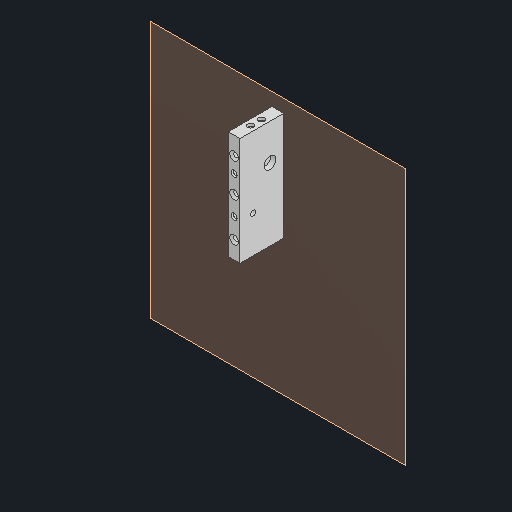
# Autodesk Inventor part: middle_gear_holder
Saved by Autodesk Inventor 2023 (Build 270158000, 158)
## iProperties
Created: 2024-04-23
Part Number: middle_gear_holder
Material: Generic
Document SubType Name: Modeling
Designer: szymo
Density: 1 g/cm^3
Appearance: Default
Author: szymo
Autodesk Inventor part; units mm, degrees
ref_plane "YZ Plane" through (0, 0, 0) normal (1, 0, 0) x (0, 1, 0)
ref_plane "XZ Plane" through (0, 0, 0) normal (0, 1, 0) x (-1, 0, 0)
ref_plane "XY Plane" through (0, 0, 0) normal (0, 0, 1) x (1, 0, 0)
ref_plane "Work Plane1" through (0, 0, 0) normal (0, 0, 1) x (1, 0, 0)
ref_plane "Work Plane2" through (-89, -40.3889, 33.5) normal (0, 0, 1) x (1, 0, 0)
sketch "Sketch1" plane through (0, 0, 0) normal (0, 0, 1) x (1, 0, 0)
  line L0 (23.5, 88.5) -> (-23.5, 88.5) projected
  line L1 (-23.5, 88.5) -> (-23.5, 36.5) projected
  line L2 (-26.5, 33.5) -> (-89, 33.5) projected
  line L3 (-89, 33.5) -> (-89, -72.5) projected
  line L4 (-89, -72.5) -> (-77, -72.5) projected
  line L5 (-74, -75.5) -> (-74, -93.5) projected
  line L6 (-74, -93.5) -> (74, -93.5) projected
  line L7 (74, -93.5) -> (74, -75.5) projected
  line L8 (77, -72.5) -> (89, -72.5) projected
  line L9 (89, -72.5) -> (89, 33.5) projected
  line L10 (89, 33.5) -> (26.5, 33.5) projected
  line L11 (23.5, 36.5) -> (23.5, 88.5) projected
  line L12 (-4.5, 81.5) -> (-4.5, 36.5) projected
  line L13 (-7.5, 33.5) -> (-13.5, 33.5) projected
  line L14 (-16.5, 36.5) -> (-16.5, 81.5) projected
  line L15 (7.5, 84.5) -> (13.5, 84.5) projected
  line L16 (16.5, 81.5) -> (16.5, 36.5) projected
  line L17 (13.5, 33.5) -> (7.5, 33.5) projected
  line L18 (4.5, 36.5) -> (4.5, 81.5) projected
  line L19 (-13.5, 84.5) -> (-7.5, 84.5) projected
  line L20 (-4.5, 88.5) -> (4.5, 88.5)
  line L21 (4.5, 88.5) -> (4.5, 5.75)
  line L22 (4.5, 5.75) -> (-4.5, 5.75)
  line L23 (-4.5, 5.75) -> (-4.5, 88.5)
  line L24 (-32.2, 4.75) -> (-59.9, 4.75)
  arc A0 (13.5, 33.5) -> (16.5, 36.5) centre (13.5, 36.5) ccw projected
  arc A1 (4.5, 36.5) -> (7.5, 33.5) centre (7.5, 36.5) ccw projected
  arc A2 (7.5, 84.5) -> (4.5, 81.5) centre (7.5, 81.5) ccw projected
  arc A3 (16.5, 81.5) -> (13.5, 84.5) centre (13.5, 81.5) ccw projected
  arc A4 (-4.5, 81.5) -> (-7.5, 84.5) centre (-7.5, 81.5) ccw projected
  arc A5 (-7.5, 33.5) -> (-4.5, 36.5) centre (-7.5, 36.5) ccw projected
  arc A6 (-16.5, 36.5) -> (-13.5, 33.5) centre (-13.5, 36.5) ccw projected
  arc A7 (-13.5, 84.5) -> (-16.5, 81.5) centre (-13.5, 81.5) ccw projected
  arc A8 (-26.5, 33.5) -> (-23.5, 36.5) centre (-26.5, 36.5) ccw projected
  arc A9 (-74, -75.5) -> (-77, -72.5) centre (-77, -75.5) ccw projected
  arc A10 (77, -72.5) -> (74, -75.5) centre (77, -75.5) ccw projected
  arc A11 (23.5, 36.5) -> (26.5, 33.5) centre (26.5, 36.5) ccw projected
  circle A12 centre (21.5, -85.5) radius 1.8 projected
  circle A13 centre (-64.5, -85.5) radius 1.8 projected
  circle A14 centre (83.4, -16.3889) radius 1.8 projected
  circle A15 centre (-83.4, -19.2889) radius 1.8 projected
  circle A16 centre (-21.5, -85.5) radius 1.8 projected
  circle A17 centre (64.5, -85.5) radius 1.8 projected
  circle A18 centre (-56.0375, 15.0937) radius 1.0065 projected
  circle A19 centre (39.125, 4.3375) radius 1.0065 projected
  circle A20 centre (-72.95, 4.275) radius 1.0065 projected
  circle A21 centre (39.125, 25.9125) radius 1.0065 projected
  circle A22 centre (72.95, 12.275) radius 1.0065 projected
  circle A23 centre (86, 30.5) radius 1.0065 projected
  circle A24 centre (-86, 30.5) radius 1.0065 projected
  circle A25 centre (-39.125, 12.3375) radius 1.0065 projected
  circle A26 centre (-72.95, 25.975) radius 1.0065 projected
  circle A27 centre (-72.95, 12.275) radius 1.0065 projected
  circle A28 centre (-39.125, 25.9125) radius 1.0065 projected
  circle A29 centre (-86, 7.75) radius 1.0065 projected
  circle A30 centre (86, 7.75) radius 1.0065 projected
  circle A31 centre (72.95, 25.975) radius 1.0065 projected
  circle A32 centre (39.125, 12.3375) radius 1.0065 projected
  circle A33 centre (-39.125, 4.3375) radius 1.0065 projected
  circle A34 centre (72.95, 4.275) radius 1.0065 projected
  circle A35 centre (56.0375, 15.125) radius 1.0065 projected
  circle A36 centre (78, -67.1725) radius 1.2295 projected
  circle A37 centre (-24.1, -73.1) radius 1.2295 projected
  circle A38 centre (24.1, -24.9) radius 1.2295 projected
  circle A39 centre (-42.5, -43.2802) radius 1.2295 projected
  circle A40 centre (-79, -42.3889) radius 1.2295 projected
  circle A41 centre (-19.5, 28.875) radius 1.2295 projected
  circle A42 centre (19.5, 9.55) radius 1.2295 projected
  circle A43 centre (19.5, 47.3) radius 1.2295 projected
  circle A44 centre (-19.5, 47.3) radius 1.2295 projected
  circle A45 centre (0, 74.7) radius 1.2295 projected
  circle A46 centre (-19.4231, 74.8077) radius 1.2295 projected
  circle A47 centre (19.5, 74.7) radius 1.2295 projected
  circle A48 centre (0, 49.05) radius 1.2295 projected
  circle A49 centre (19.5, 28.875) radius 1.2295 projected
  circle A50 centre (0, 19.125) radius 1.2295 projected
  circle A51 centre (-19.5, 9.55) radius 1.2295 projected
  circle A52 centre (-78, -67.1725) radius 1.2295 projected
  circle A53 centre (-24.1, -24.9) radius 1.2295 projected
  circle A54 centre (24.1, -73.1) radius 1.2295 projected
  circle A55 centre (42.5, -42.7745) radius 1.2295 projected
  circle A56 centre (79, -42.3889) radius 1.2295 projected
  line L25 (-71, -46.1649) -> (-65.2254, -46.1649) projected
  arc A57 (-63.098, -51.2802) -> (-65.2254, -46.1649) centre (-65.2254, -49.1649) ccw projected
  line L26 (-63.098, -51.2802) -> (-68.8726, -57.0881) projected
  arc A58 (-74, -54.9729) -> (-68.8726, -57.0881) centre (-71, -54.9729) ccw projected
  line L27 (-74, -54.9729) -> (-74, -49.1649) projected
  arc A59 (-71, -46.1649) -> (-74, -49.1649) centre (-71, -49.1649) ccw projected
  line L28 (-18.5, -8.7315) -> (-18.5, -4.7315) projected
  arc A60 (-15.5, -1.7315) -> (-18.5, -4.7315) centre (-15.5, -4.7315) ccw projected
  line L29 (-15.5, -1.7315) -> (-8.5, -1.7315) projected
  arc A61 (-5.5, -4.7315) -> (-8.5, -1.7315) centre (-8.5, -4.7315) ccw projected
  line L30 (-5.5, -4.7315) -> (-5.5, -8.7315) projected
  arc A62 (-8.5, -11.7315) -> (-5.5, -8.7315) centre (-8.5, -8.7315) ccw projected
  line L31 (-8.5, -11.7315) -> (-15.5, -11.7315) projected
  arc A63 (-18.5, -8.7315) -> (-15.5, -11.7315) centre (-15.5, -8.7315) ccw projected
  line L32 (-62.5563, -19.7315) -> (-38.9437, -19.7315) projected
  arc A64 (-36.8163, -24.8467) -> (-38.9437, -19.7315) centre (-38.9437, -22.7315) ccw projected
  line L33 (-36.8163, -24.8467) -> (-48.6226, -36.7211) projected
  arc A65 (-52.8774, -36.7211) -> (-48.6226, -36.7211) centre (-50.75, -34.6059) ccw projected
  line L34 (-52.8774, -36.7211) -> (-64.6837, -24.8467) projected
  arc A66 (-62.5563, -19.7315) -> (-64.6837, -24.8467) centre (-62.5563, -22.7315) ccw projected
  line L35 (27.5, -54.9729) -> (27.5, -49.1649) projected
  arc A67 (30.5, -46.1649) -> (27.5, -49.1649) centre (30.5, -49.1649) ccw projected
  line L36 (30.5, -46.1649) -> (36.2746, -46.1649) projected
  arc A68 (38.402, -51.2802) -> (36.2746, -46.1649) centre (36.2746, -49.1649) ccw projected
  line L37 (38.402, -51.2802) -> (32.6274, -57.0881) projected
  arc A69 (27.5, -54.9729) -> (32.6274, -57.0881) centre (30.5, -54.9729) ccw projected
  line L38 (10.6273, -24.5614) -> (1.8773, -35.9288) projected
  arc A70 (-2.8773, -35.9288) -> (1.8773, -35.9288) centre (-0.5, -34.0989) ccw projected
  line L39 (-2.8773, -35.9288) -> (-11.6273, -24.5614) projected
  arc A71 (-9.25, -19.7315) -> (-11.6273, -24.5614) centre (-9.25, -22.7315) ccw projected
  line L40 (-9.25, -19.7315) -> (8.25, -19.7315) projected
  arc A72 (10.6273, -24.5614) -> (8.25, -19.7315) centre (8.25, -22.7315) ccw projected
  line L41 (-32.6274, -57.0881) -> (-38.402, -51.2802) projected
  arc A73 (-36.2746, -46.1649) -> (-38.402, -51.2802) centre (-36.2746, -49.1649) ccw projected
  line L42 (-36.2746, -46.1649) -> (-30.5, -46.1649) projected
  arc A74 (-27.5, -49.1649) -> (-30.5, -46.1649) centre (-30.5, -49.1649) ccw projected
  line L43 (-27.5, -49.1649) -> (-27.5, -54.9729) projected
  arc A75 (-32.6274, -57.0881) -> (-27.5, -54.9729) centre (-30.5, -54.9729) ccw projected
  spline S0 degree 3 poles (58.9, 23.725) (58.9, 24.1577) (58.9848, 24.5947) (59.3384, 25.472) (59.607, 25.8253) (60.2494, 26.5053) (60.6866, 26.7292) (61.3735, 27.0327) (61.8092, 27.1082) (62.6877, 27.1429) (63.1304, 27.039) (63.9304, 26.7523) (64.2888, 26.5005) (64.9284, 25.9459) (65.1766, 25.5677) (65.4139, 25.1026) (65.5281, 24.8465) (65.6683, 24.2527) (65.7, 23.9883) (65.7, 23.725) knots 0 0 0 0 0.129822 0.129822 0.282673 0.282673 0.568071 0.568071 1.093785 1.093785 1.85316 1.85316 2.989395 2.989395 4.855548 4.855548 5.876131 5.876131 6.645928 6.645928 6.645928 6.645928 projected
  line L44 (65.7, 23.725) -> (65.7, 14.525) projected
  spline S1 degree 3 poles (65.7, 14.525) (65.7, 14.0923) (65.6152, 13.6553) (65.2616, 12.778) (64.993, 12.4247) (64.3506, 11.7447) (63.9134, 11.5208) (63.2265, 11.2173) (62.7908, 11.1418) (61.9123, 11.1071) (61.4696, 11.211) (60.6696, 11.4977) (60.3112, 11.7495) (59.6716, 12.3041) (59.4234, 12.6823) (59.1861, 13.1474) (59.0719, 13.4035) (58.9317, 13.9973) (58.9, 14.2617) (58.9, 14.525) knots 0 0 0 0 0.129822 0.129822 0.282673 0.282673 0.568071 0.568071 1.093785 1.093785 1.85316 1.85316 2.989395 2.989395 4.855548 4.855548 5.876131 5.876131 6.645928 6.645928 6.645928 6.645928 projected
  line L45 (58.9, 14.525) -> (58.9, 23.725) projected
  line L46 (-36.734, -33.2737) -> (-32.6274, -29.1434) projected
  arc A76 (-27.5, -31.2586) -> (-32.6274, -29.1434) centre (-30.5, -31.2586) ccw projected
  line L47 (-27.5, -31.2586) -> (-27.5, -35.3889) projected
  arc A77 (-30.5, -38.3889) -> (-27.5, -35.3889) centre (-30.5, -35.3889) ccw projected
  line L48 (-30.5, -38.3889) -> (-34.6065, -38.3889) projected
  arc A78 (-36.734, -33.2737) -> (-34.6065, -38.3889) centre (-34.6065, -35.3889) ccw projected
  line L49 (12.1227, -55.4157) -> (2.6549, -43.1158) projected
  line L50 (2.6549, -43.1158) -> (12.1227, -30.8158) projected
  arc A79 (17.5, -32.6457) -> (12.1227, -30.8158) centre (14.5, -32.6457) ccw projected
  line L51 (17.5, -32.6457) -> (17.5, -53.5858) projected
  arc A80 (12.1227, -55.4157) -> (17.5, -53.5858) centre (14.5, -53.5858) ccw projected
  line L52 (74, -31.2586) -> (74, -36.3889) projected
  arc A81 (71, -39.3889) -> (74, -36.3889) centre (71, -36.3889) ccw projected
  line L53 (71, -39.3889) -> (65.8992, -39.3889) projected
  arc A82 (63.7718, -34.2737) -> (65.8992, -39.3889) centre (65.8992, -36.3889) ccw projected
  line L54 (63.7718, -34.2737) -> (68.8726, -29.1434) projected
  arc A83 (74, -31.2586) -> (68.8726, -29.1434) centre (71, -31.2586) ccw projected
  line L55 (-27.5, -4.7315) -> (-27.5, -8.7315) projected
  arc A84 (-30.5, -11.7315) -> (-27.5, -8.7315) centre (-30.5, -8.7315) ccw projected
  line L56 (-30.5, -11.7315) -> (-42.75, -11.7315) projected
  arc A85 (-45.75, -8.7315) -> (-42.75, -11.7315) centre (-42.75, -8.7315) ccw projected
  line L57 (-45.75, -8.7315) -> (-45.75, -4.7315) projected
  arc A86 (-42.75, -1.7315) -> (-45.75, -4.7315) centre (-42.75, -4.7315) ccw projected
  line L58 (-42.75, -1.7315) -> (-30.5, -1.7315) projected
  arc A87 (-27.5, -4.7315) -> (-30.5, -1.7315) centre (-30.5, -4.7315) ccw projected
  line L59 (74, -4.7315) -> (74, -8.7315) projected
  arc A88 (71, -11.7315) -> (74, -8.7315) centre (71, -8.7315) ccw projected
  line L60 (71, -11.7315) -> (58.75, -11.7315) projected
  arc A89 (55.75, -8.7315) -> (58.75, -11.7315) centre (58.75, -8.7315) ccw projected
  line L61 (55.75, -8.7315) -> (55.75, -4.7315) projected
  arc A90 (58.75, -1.7315) -> (55.75, -4.7315) centre (58.75, -4.7315) ccw projected
  line L62 (58.75, -1.7315) -> (71, -1.7315) projected
  arc A91 (74, -4.7315) -> (71, -1.7315) centre (71, -4.7315) ccw projected
  line L63 (62.5563, -66.5) -> (38.9437, -66.5) projected
  arc A92 (36.8163, -61.3848) -> (38.9437, -66.5) centre (38.9437, -63.5) ccw projected
  line L64 (36.8163, -61.3848) -> (48.6226, -49.5104) projected
  arc A93 (52.8774, -49.5104) -> (48.6226, -49.5104) centre (50.75, -51.6256) ccw projected
  line L65 (52.8774, -49.5104) -> (64.6837, -61.3848) projected
  arc A94 (62.5563, -66.5) -> (64.6837, -61.3848) centre (62.5563, -63.5) ccw projected
  line L66 (17.5, -4.7315) -> (17.5, -8.7315) projected
  arc A95 (14.5, -11.7315) -> (17.5, -8.7315) centre (14.5, -8.7315) ccw projected
  line L67 (14.5, -11.7315) -> (7.5, -11.7315) projected
  arc A96 (4.5, -8.7315) -> (7.5, -11.7315) centre (7.5, -8.7315) ccw projected
  line L68 (4.5, -8.7315) -> (4.5, -4.7315) projected
  arc A97 (7.5, -1.7315) -> (4.5, -4.7315) centre (7.5, -4.7315) ccw projected
  line L69 (7.5, -1.7315) -> (14.5, -1.7315) projected
  arc A98 (17.5, -4.7315) -> (14.5, -1.7315) centre (14.5, -4.7315) ccw projected
  line L70 (38.9437, -19.7315) -> (62.5563, -19.7315) projected
  arc A99 (64.6837, -24.8467) -> (62.5563, -19.7315) centre (62.5563, -22.7315) ccw projected
  line L71 (64.6837, -24.8467) -> (52.8774, -36.7211) projected
  arc A100 (48.6226, -36.7211) -> (52.8774, -36.7211) centre (50.75, -34.6059) ccw projected
  line L72 (48.6226, -36.7211) -> (36.8163, -24.8467) projected
  arc A101 (38.9437, -19.7315) -> (36.8163, -24.8467) centre (38.9437, -22.7315) ccw projected
  line L73 (-18.5, -53.5858) -> (-18.5, -32.6457) projected
  arc A102 (-13.1227, -30.8158) -> (-18.5, -32.6457) centre (-15.5, -32.6457) ccw projected
  line L74 (-13.1227, -30.8158) -> (-3.6549, -43.1158) projected
  line L75 (-3.6549, -43.1158) -> (-13.1227, -55.4157) projected
  arc A103 (-18.5, -53.5858) -> (-13.1227, -55.4157) centre (-15.5, -53.5858) ccw projected
  line L76 (-38.9437, -66.5) -> (-62.5563, -66.5) projected
  arc A104 (-64.6837, -61.3848) -> (-62.5563, -66.5) centre (-62.5563, -63.5) ccw projected
  line L77 (-64.6837, -61.3848) -> (-52.8774, -49.5104) projected
  arc A105 (-48.6226, -49.5104) -> (-52.8774, -49.5104) centre (-50.75, -51.6256) ccw projected
  line L78 (-48.6226, -49.5104) -> (-36.8163, -61.3848) projected
  arc A106 (-38.9437, -66.5) -> (-36.8163, -61.3848) centre (-38.9437, -63.5) ccw projected
  line L79 (-58.9, 23.725) -> (-58.9, 14.525) projected
  spline S2 degree 3 poles (-58.9, 14.525) (-58.9, 14.0923) (-58.9848, 13.6553) (-59.3384, 12.778) (-59.607, 12.4247) (-60.2494, 11.7447) (-60.6866, 11.5208) (-61.3735, 11.2173) (-61.8092, 11.1418) (-62.6877, 11.1071) (-63.1304, 11.211) (-63.9304, 11.4977) (-64.2888, 11.7495) (-64.9284, 12.3041) (-65.1766, 12.6823) (-65.4139, 13.1474) (-65.5281, 13.4035) (-65.6683, 13.9973) (-65.7, 14.2617) (-65.7, 14.525) knots 0 0 0 0 0.129822 0.129822 0.282673 0.282673 0.568071 0.568071 1.093785 1.093785 1.85316 1.85316 2.989395 2.989395 4.855548 4.855548 5.876131 5.876131 6.645928 6.645928 6.645928 6.645928 projected
  line L80 (-65.7, 14.525) -> (-65.7, 23.725) projected
  spline S3 degree 3 poles (-65.7, 23.725) (-65.7, 24.1577) (-65.6152, 24.5947) (-65.2616, 25.472) (-64.993, 25.8253) (-64.3506, 26.5053) (-63.9134, 26.7292) (-63.2265, 27.0327) (-62.7908, 27.1082) (-61.9123, 27.1429) (-61.4696, 27.039) (-60.6696, 26.7523) (-60.3112, 26.5005) (-59.6716, 25.9459) (-59.4234, 25.5677) (-59.1861, 25.1026) (-59.0719, 24.8465) (-58.9317, 24.2527) (-58.9, 23.9883) (-58.9, 23.725) knots 0 0 0 0 0.129822 0.129822 0.282673 0.282673 0.568071 0.568071 1.093785 1.093785 1.85316 1.85316 2.989395 2.989395 4.855548 4.855548 5.876131 5.876131 6.645928 6.645928 6.645928 6.645928 projected
  line L81 (-74, -35.3889) -> (-74, -31.2586) projected
  arc A107 (-68.8726, -29.1434) -> (-74, -31.2586) centre (-71, -31.2586) ccw projected
  line L82 (-68.8726, -29.1434) -> (-64.766, -33.2737) projected
  arc A108 (-66.8935, -38.3889) -> (-64.766, -33.2737) centre (-66.8935, -35.3889) ccw projected
  line L83 (-66.8935, -38.3889) -> (-71, -38.3889) projected
  arc A109 (-74, -35.3889) -> (-71, -38.3889) centre (-71, -35.3889) ccw projected
  line L84 (8.25, -66.5) -> (-9.25, -66.5) projected
  arc A110 (-11.6273, -61.6701) -> (-9.25, -66.5) centre (-9.25, -63.5) ccw projected
  line L85 (-11.6273, -61.6701) -> (-2.8773, -50.3027) projected
  arc A111 (1.8773, -50.3027) -> (-2.8773, -50.3027) centre (-0.5, -52.1326) ccw projected
  line L86 (1.8773, -50.3027) -> (10.6273, -61.6701) projected
  arc A112 (8.25, -66.5) -> (10.6273, -61.6701) centre (8.25, -63.5) ccw projected
  line L87 (68.8726, -57.0881) -> (63.098, -51.2802) projected
  arc A113 (65.2254, -46.1649) -> (63.098, -51.2802) centre (65.2254, -49.1649) ccw projected
  line L88 (65.2254, -46.1649) -> (71, -46.1649) projected
  arc A114 (74, -49.1649) -> (71, -46.1649) centre (71, -49.1649) ccw projected
  line L89 (74, -49.1649) -> (74, -54.9729) projected
  arc A115 (68.8726, -57.0881) -> (74, -54.9729) centre (71, -54.9729) ccw projected
  line L90 (-74, -8.7315) -> (-74, -4.7315) projected
  arc A116 (-71, -1.7315) -> (-74, -4.7315) centre (-71, -4.7315) ccw projected
  line L91 (-71, -1.7315) -> (-58.75, -1.7315) projected
  arc A117 (-55.75, -4.7315) -> (-58.75, -1.7315) centre (-58.75, -4.7315) ccw projected
  line L92 (-55.75, -4.7315) -> (-55.75, -8.7315) projected
  arc A118 (-58.75, -11.7315) -> (-55.75, -8.7315) centre (-58.75, -8.7315) ccw projected
  line L93 (-58.75, -11.7315) -> (-71, -11.7315) projected
  arc A119 (-74, -8.7315) -> (-71, -11.7315) centre (-71, -8.7315) ccw projected
  line L94 (27.5, -8.7315) -> (27.5, -4.7315) projected
  arc A120 (30.5, -1.7315) -> (27.5, -4.7315) centre (30.5, -4.7315) ccw projected
  line L95 (30.5, -1.7315) -> (42.75, -1.7315) projected
  arc A121 (45.75, -4.7315) -> (42.75, -1.7315) centre (42.75, -4.7315) ccw projected
  line L96 (45.75, -4.7315) -> (45.75, -8.7315) projected
  arc A122 (42.75, -11.7315) -> (45.75, -8.7315) centre (42.75, -8.7315) ccw projected
  line L97 (42.75, -11.7315) -> (30.5, -11.7315) projected
  arc A123 (27.5, -8.7315) -> (30.5, -11.7315) centre (30.5, -8.7315) ccw projected
  line L98 (32.6274, -29.1434) -> (37.7282, -34.2737) projected
  arc A124 (35.6008, -39.3889) -> (37.7282, -34.2737) centre (35.6008, -36.3889) ccw projected
  line L99 (35.6008, -39.3889) -> (30.5, -39.3889) projected
  arc A125 (27.5, -36.3889) -> (30.5, -39.3889) centre (30.5, -36.3889) ccw projected
  line L100 (27.5, -36.3889) -> (27.5, -31.2586) projected
  arc A126 (32.6274, -29.1434) -> (27.5, -31.2586) centre (30.5, -31.2586) ccw projected
  point P0 (0, 0)
  point P1 (-4.5, 81.5)
  point P2 (-4.5, 36.5)
  point P3 (7.5, 81.5)
  point P4 (13.5, 81.5)
  point P5 (-7.5, 81.5)
  point P6 (-13.5, 81.5)
  dimension "d41" = 1
  constraints: 10 end point, 2 collinear, 2 horizontal, 2 parallel, 1 perpendicular, 1 point on line, 2 other
  measures "d41" distance between parallel lines of L22 L24
extrude "Extrusion1" add sketch "Sketch1" along normal up to surface (33.5 mm away) contours L21 L18 L22 L23 L12 L0 | A45 | A48 | A50
sketch "Sketch2" plane through (4.5, 5.75, 0) normal (1, 0, 0) x (0, 0, -1)
  circle A0 centre (-23.4363, 28.1825) radius 2 projected
  point P0 (0, -5.75)
extrude "Extrusion2" cut sketch "Sketch2" against normal blind 10
sketch "Sketch3" plane through (4.5, 5.75, 0) normal (1, 0, 0) x (0, 0, -1)
  circle A0 centre (-10.5, 55.25) radius 4.5 projected
  point P0 (0, -5.75)
extrude "Extrusion3" cut sketch "Sketch3" against normal blind 4
sketch "Sketch4" plane through (-4.5, 5.75, 0) normal (-1, 0, 0) x (0, 0, 1)
  circle A0 centre (10.5, 55.25) radius 4.5 projected
  point P0 (0, -5.75)
extrude "Extrusion4" cut sketch "Sketch4" against normal blind 4
sketch "Sketch5" plane through (-4.5, 5.75, 33.5) normal (0, 0, 1) x (1, 0, 0)
  line L0 (5, 59.75) -> (5, 50.75) projected
  line L1 (4, 50.75) -> (4, 59.75) projected
  line L2 (9, 26.1825) -> (0, 26.1825) projected
  line L3 (9, 30.1825) -> (0, 30.1825) projected
  line L4 (17, 78.15) -> (-8, 78.15)
  line L5 (-8, 35.85) -> (17, 35.85)
  line L6 (9, 82.75) -> (9, 0) projected
  line L7 (0, 50.75) -> (0, 59.75) projected
  line L8 (9, 35.85) -> (0, 35.85)
  line L9 (0, 35.85) -> (0, 50.75)
  line L10 (0, 50.75) -> (9, 50.75)
  line L11 (9, 50.75) -> (9, 35.85)
  line L12 (0, 0) -> (0, 82.75) projected
  line L13 (9, 78.15) -> (0, 78.15)
  line L14 (0, 78.15) -> (0, 59.75)
  line L15 (0, 59.75) -> (9, 59.75)
  line L16 (9, 59.75) -> (9, 78.15)
  line L17 (-18, 6.625) -> (-18, 20.125) projected
  line L18 (-18, 13.375) -> (27, 13.375)
  line L19 (9, 35.85) -> (0, 50.75)
  line L20 (9, 59.75) -> (9, 50.75) projected
  line L21 (0, 35.85) -> (9, 50.75)
  line L22 (9, 59.75) -> (0, 78.15)
  line L23 (0, 59.75) -> (9, 78.15)
  point P0 (4.5, -5.75)
  point P1 (4.5, 13.375)
  point P2 (4.5, 43.3)
  point P3 (4.5, 68.95)
  dimension "d9" = 4.5
  dimension "d10" = 4.5
  constraints: 30 end point, 5 horizontal, 5 point on line, 4 midpoint, 4 parallel, 2 perpendicular, 4 other
  measures "d9" distance from line of L6 point (4.5, 13.375)
  measures "d10" distance from line of point (4.5, 13.375) L12
hole "Hole1" at (0, 19.125, 33.5) at (0, 49.05, 33.5) at (0, 74.7, 33.5) direction (0, 0, -1) diameter 3.6 end through all countersink diameter 6.6 countersink angle 90 clearance for "Countersunk Flat Head Screw ISO 2009/7046" size "M3" standard "ISO"
sketch "Sketch6" plane through (-4.5, 5.75, 0) normal (0, -1, 0) x (1, 0, 0)
  line L0 (9, 33.5) -> (0, 33.5) projected
  line L1 (0, 0) -> (0, 33.5) projected
  line L2 (0, 0) -> (9, 0) projected
  line L3 (9, 0) -> (9, 33.5) projected
  line L4 (0, 16.75) -> (9, 16.75)
  line L5 (9, 16.75) -> (0, 33.5)
  line L6 (9, 33.5) -> (0, 16.75)
  line L7 (0, 16.75) -> (9, 0)
  line L8 (9, 16.75) -> (0, 0)
  point P0 (4.5, 0)
  point P1 (4.5, 8.375)
  point P2 (4.5, 25.125)
  constraints: 10 end point, 4 midpoint, 2 parallel
hole "Hole2" at (0, 5.75, 8.375) at (0, 5.75, 25.125) direction (0, 1, 0) diameter 4 depth 6.6 counterbore diameter 5 counterbore depth 2
sketch "Sketch7" plane through (-4.5, 88.5, 0) normal (0, 1, 0) x (1, 0, 0)
  line L0 (0, -33.5) -> (9, -33.5) projected
  line L1 (0, -33.5) -> (9, -33.5) projected
  line L2 (9, 0) -> (9, -33.5) projected
  line L3 (9, 0) -> (0, 0) projected
  line L4 (0, 0) -> (0, -33.5) projected
  line L5 (-8, -1.4) -> (-8, -6.6) projected
  line L6 (-8, -32.1) -> (-8, -26.9) projected
  line L7 (17, -32.1) -> (17, -26.9) projected
  line L8 (17, -1.4) -> (17, -6.6) projected
  line L9 (17, -32.1) -> (-8, -32.1)
  line L10 (-8, -32.1) -> (-8, -26.9)
  line L11 (-8, -26.9) -> (17, -26.9)
  line L12 (17, -26.9) -> (17, -32.1)
  line L13 (-8, -6.6) -> (17, -6.6)
  line L14 (17, -6.6) -> (17, -1.4)
  line L15 (17, -1.4) -> (-8, -1.4)
  line L16 (-8, -1.4) -> (-8, -6.6)
  line L17 (17, -6.6) -> (-8, -6.6)
  line L18 (-8, -6.6) -> (-8, -8.6)
  line L19 (-8, -8.6) -> (17, -8.6)
  line L20 (17, -8.6) -> (17, -6.6)
  line L21 (-8, -26.9) -> (17, -26.9)
  line L22 (17, -26.9) -> (17, -24.9)
  line L23 (17, -24.9) -> (-8, -24.9)
  line L24 (-8, -24.9) -> (-8, -26.9)
  line L25 (9, 0) -> (9, -33.5) projected
  line L26 (9, -16.75) -> (0, -16.75)
  line L27 (0, 0) -> (0, -33.5) projected
  line L28 (9, -24.9) -> (0, -16.75)
  line L29 (9, -8.6) -> (0, -16.75)
  line L30 (0, -8.6) -> (9, -16.75)
  line L31 (9, -16.75) -> (0, -24.9)
  point P0 (4.5, 0)
  point P1 (4.5, -20.825)
  point P2 (4.5, -12.675)
  dimension "d25" = 2
  dimension "d26" = 2
  constraints: 42 end point, 10 point on line, 8 parallel, 5 midpoint, 4 horizontal, 4 perpendicular
  measures "d25" distance of L18.end L17.end
  measures "d26" distance of L22.end L21.end
hole "Hole3" at (0, 88.5, 20.825) at (0, 88.5, 12.675) direction (0, -1, 0) diameter 4 depth 6.5 counterbore diameter 4.6 counterbore depth 2
sketch "Sketch8" plane through (-4.5, 5.75, 33.5) normal (0, 0, 1) x (1, 0, 0)
  line L0 (26, 27.2497) -> (-17, 27.2497)
  line L1 (26, 31.2497) -> (-17, 31.2497)
  line L2 (4, 52.75) -> (-1, 52.75)
  line L3 (4, 61.75) -> (-1, 61.75)
  line L4 (10, 61.75) -> (5, 61.75)
  line L5 (9, 50.75) -> (5, 50.75) projected
  line L6 (0, 0) -> (0, 82.75) projected
  line L7 (9, 52.75) -> (0, 52.75)
  line L8 (0, 52.75) -> (0, 61.75)
  line L9 (0, 61.75) -> (9, 61.75)
  line L10 (9, 61.75) -> (9, 50.75)
  line L11 (9, 26.1825) -> (0, 26.1825) projected
  line L12 (0, 31.2497) -> (9, 31.2497)
  line L13 (9, 31.2497) -> (9, 26.1825)
  line L14 (9, 26.1825) -> (0, 26.1825)
  line L15 (0, 26.1825) -> (0, 31.2497)
  line L16 (9, 26.1825) -> (0, 31.2497)
  line L17 (0, 26.1825) -> (9, 31.2497)
  line L18 (10, 51.75) -> (0, 61.75)
  line L19 (0, 52.75) -> (9, 61.75)
  point P0 (4.5, -5.75)
  point P1 (4.5, 28.7161)
  point P2 (4.5, 57.25)
  constraints: 34 end point, 7 horizontal, 6 point on line, 4 parallel, 3 perpendicular, 2 midpoint, 10 other
hole "Hole4" at (0, 34.4661, 33.5) at (0, 63, 33.5) direction (0, 0, -1) diameter 4 depth 6 counterbore diameter 4.6 counterbore depth 1.5
equation "\"d9\" = d10"
body "Solid1"
